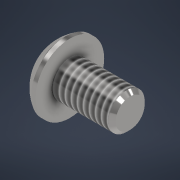
# Autodesk Inventor part: bolt_2_5mm
Saved by Autodesk Inventor 2021.3 (Build 253353000, 353)
## iProperties
Created: 2021-10-17
Part Number: bolt_2_5mm
Material: Steel, Mild, Welded
Document SubType Name: Modeling
Designer: ASUS
Density: 7.85 g/cm^3
Appearance: Steel - Polished
Author: ASUS
Autodesk Inventor part; units mm, degrees
ref_plane "YZ Plane" through (0, 0, 0) normal (1, 0, 0) x (0, 1, 0)
ref_plane "XZ Plane" through (0, 0, 0) normal (0, 1, 0) x (-1, 0, 0)
ref_plane "XY Plane" through (0, 0, 0) normal (0, 0, 1) x (1, 0, 0)
sketch "Sketch1" plane through (0, 0, 0) normal (0, 0, 1) x (1, 0, 0)
  line L0 (-16.019, 0) -> (-11.019, 0)
  line L1 (-16.019, 1.5) -> (-11.319, 1.5)
  line L2 (-16.019, 0) -> (-16.019, 2.85)
  line L3 (-17.669, 0) -> (-17.669, 1.425)
  line L4 (-11.019, 1.2) -> (-11.019, 0)
  line L5 (-16.369, 0) -> (-16.369, 2.85)
  line L6 (-16.019, 2.85) -> (-16.369, 2.85)
  arc A0 (-16.369, 2.85) -> (-17.669, 1.425) centre (-14.6489, -0.0247) ccw
  line L7 (-11.319, 1.5) -> (-11.019, 1.2)
  line L8 (-16.019, 0) -> (-17.669, 0)
  point P0 (0, 0)
  point P1 (-11.019, 1.5)
  dimension "d0" = 5
  dimension "d1" = 1.5
  dimension "d2" = 2.85
  dimension "d3" = 1.425
  dimension "d4" = 1.65
  dimension "d5" = 2.85
  dimension "d6" = 0.35
  dimension "d7" = 3.35
  dimension "d8" = 0.3
  dimension "d9" = 45
  constraints: 18 end point, 4 vertical, 3 horizontal, 2 point on circle, 2 point on line, 1 centre point, 1 parallel
  measures "d0" distance of L0.start L0.end
  measures "d1" distance between parallel lines of L0 L1
  measures "d2" distance of L0.start L2.end
  measures "d3" distance of L3.start L3.end
  measures "d4" distance between parallel lines of L2 L3
  measures "d5" distance of L5.start L5.end
  measures "d6" distance between parallel lines of L5 L2
  measures "d7" radius of A0
  measures "d8" distance of L1.end point (-11.019, 1.5)
  measures "d9" angle of L1 L7
revolve "Revolution1" add sketch "Sketch1" angle 360 about axis through (-16.019, 0, 0) along (1, 0, 0)
sketch "Sketch2" plane through (-17.669, 0, 0) normal (-1, 0, 0) x (0, 0, 1)
  line L0 (-1, 0) -> (-0.5, 0.866)
  line L1 (-0.5, 0.866) -> (0.5, 0.866)
  line L2 (0.5, 0.866) -> (1, 0)
  line L3 (1, 0) -> (0.5, -0.866)
  line L4 (0.5, -0.866) -> (-0.5, -0.866)
  line L5 (-0.5, -0.866) -> (-1, 0)
  point P0 (0, 0)
  point P1 (0, 0)
  dimension "d11" = 2
  constraints: 12 end point, 1 coincident, 13 other
  measures "d11" distance of L2.end L0.start
extrude "Extrusion1" cut sketch "Sketch2" against normal blind 1
thread "Thread1" size "M3x0.5" class "6g" standard "ANSI Metric M Profile" full length
body "Solid1"
